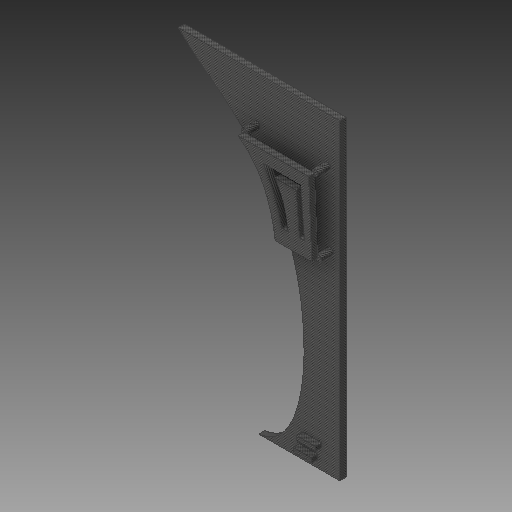
# Autodesk Inventor part: Part2 new side frame
Saved by Autodesk Inventor 2018 (Build 220112000, 112)
## iProperties
Created: 2021-03-13
Part Number: Part2 new side frame
Material: CFRP
Document SubType Name: Modeling
Designer: Abhig
Density: 1.43 g/cm^3
Appearance: Carbon Fiber
Author: Abhig
Autodesk Inventor part; units mm, degrees
ref_plane "YZ Plane" through (0, 0, 0) normal (1, 0, 0) x (0, 1, 0)
ref_plane "XZ Plane" through (0, 0, 0) normal (0, 1, 0) x (-1, 0, 0)
ref_plane "XY Plane" through (0, 0, 0) normal (0, 0, 1) x (1, 0, 0)
sketch "Sketch1" plane through (0, 0, 0) normal (0, 0, 1) x (1, 0, 0)
  line L0 (0, 226.8926) -> (200, 226.8926)
  line L1 (200, 226.8926) -> (200, -273.1074)
  line L2 (200, -273.1074) -> (70.0106, -273.1074)
  spline S0 degree 4 poles (0, 177.3413) (126.203, 79.0594) (154.2664, -10.2822) (176.0066, -260.8084) (70.0106, -273.1074) knots 0 0 0 0 0 1 1 1 1 1
  spline S1 degree 2 poles (0, 177.3413) (-36.5043, 204.7595) (-58.7785, 226.8926) knots 0 0 0 1 1 1
  line L3 (-58.7785, 226.8926) -> (0, 226.8926)
  point P0 (0, 0)
  point P1 (99.9997, 63.7426)
  point P2 (140.6791, -78.917)
  point P3 (126.8096, -220.2554)
  point P4 (-35.664, 205.7436)
  constraints: 8 end point, 2 horizontal, 1 parallel, 1 perpendicular, 10 other
extrude "Extrusion1" add sketch "Sketch1" along normal blind 10
sketch "Sketch2" plane through (0, 0, 10) normal (0, 0, 1) x (1, 0, 0)
  circle A0 centre (66.8612, 154.6625) radius 5
  circle A1 centre (180.0109, 154.6625) radius 5
  circle A2 centre (185.0109, 38.5738) radius 5
  circle A3 centre (126.375, 38.5738) radius 5
  point P0 (0, 0)
  dimension "d5" = 10
  dimension "d6" = 10
  dimension "d7" = 10
  dimension "d8" = 10
  constraints: 4 centre point
  measures "d5" diameter of A0
  measures "d6" diameter of A1
  measures "d7" diameter of A2
  measures "d8" diameter of A3
extrude "Extrusion2" add sketch "Sketch2" along normal blind 20
sketch "Sketch3" plane through (180.0109, 154.6625, 30) normal (0, 0, 1) x (1, 0, 0)
  circle A0 centre (-113.1497, 0) radius 5 projected
  circle A1 centre (0, 0) radius 5 projected
  line L0 (-113.1497, 0) -> (0, 0)
  circle A2 centre (5, -116.0887) radius 5 projected
  line L1 (0, 0) -> (5, -116.0887)
  circle A3 centre (-53.6359, -116.0887) radius 5 projected
  line L2 (5, -116.0887) -> (-53.6359, -116.0887)
  spline S0 degree 2 poles (-113.1497, 0) (-63.3738, -35.791) (-53.6359, -116.0887) knots 0 0 0 1 1 1
  point P0 (-180.0109, -154.6625)
  point P1 (-75.6781, -42.6148)
  constraints: 6 end point, 1 horizontal, 3 other
extrude "Extrusion3" add sketch "Sketch3" along normal blind 10 contours L0 A1 L1 A2 L2 A3 S0 A0 | A0 S0 L0 | L0 L1 A1 | A3 L2 S0 | L1 L2 A2 picked at (-110.3004, -1.6927) picked at (-1.6834, -2.8514) picked at (-53.6623, -112.78) picked at (1.7062, -115.7278)
sketch "Sketch4" plane through (180.0109, 154.6625, 40) normal (0, 0, 1) x (1, 0, 0)
  line L0 (-72.7391, -18.3685) -> (-12.7391, -18.3685)
  line L1 (-12.7391, -18.3685) -> (-6.5901, -92.1125)
  spline S0 degree 2 poles (-72.7391, -18.3685) (-51.5746, -50.5042) (-42.859, -93.2077) knots 0 0 0 1 1 1
  line L2 (-14.6388, -92.7837) -> (-19.9394, -29.2142)
  line L3 (-19.9394, -29.2142) -> (-55.1054, -29.2142)
  spline S1 degree 2 poles (-55.1054, -29.2142) (-38.2895, -49.2242) (-32.7381, -93.2077) knots 0 0 0 1 1 1
  line L4 (-42.859, -93.2077) -> (-32.7381, -93.2077)
  line L5 (-14.6388, -92.7837) -> (-6.5901, -92.1125)
  point P0 (-180.0109, -154.6625)
  point P1 (-55.1635, -51.9626)
  point P2 (-42.687, -50.9557)
  dimension "d13" = 60
  dimension "d14" = 74
  constraints: 12 end point, 3 horizontal, 1 perpendicular, 6 other
  measures "d13" distance of L0.start L0.end
  measures "d14" distance of L0.end L1.end
extrude "Extrusion4" cut sketch "Sketch4" against normal blind 10
sketch "Sketch6" plane through (0, 0, 10) normal (0, 0, 1) x (1, 0, 0)
  line L0 (135.0053, -253.8522) -> (165.0053, -253.8522)
  line L1 (165.0053, -253.8522) -> (165.0053, -260.8522)
  line L2 (165.0053, -260.8522) -> (135.0053, -260.8522)
  line L3 (135.0053, -260.8522) -> (135.0053, -253.8522)
  line L4 (141.0698, -234.749) -> (171.0698, -234.749)
  line L5 (171.0698, -234.749) -> (171.0698, -241.749)
  line L6 (171.0698, -241.749) -> (141.0698, -241.749)
  line L7 (141.0698, -241.749) -> (141.0698, -234.749)
  point P0 (0, 0)
  dimension "d22" = 30
  dimension "d23" = 7
  dimension "d24" = 30
  dimension "d25" = 7
  constraints: 16 end point, 4 parallel, 2 horizontal, 2 perpendicular
  measures "d22" distance of L1.end L2.end
  measures "d23" distance of L0.end L1.end
  measures "d24" distance of L5.end L6.end
  measures "d25" distance of L4.end L5.end
extrude "Extrusion6" add sketch "Sketch6" along normal blind 10
sketch "Sketch8" plane through (0, 0, 0) normal (0, 0, -1) x (-1, 0, 0)
  circle A0 centre (-180.0109, 154.6625) radius 5 projected
  circle A1 centre (-180.0109, 154.6625) radius 5
  line L0 (-180.0109, 154.6625) -> (-154.3956, -221.4322) construction
  circle A2 centre (-154.3956, -221.4322) radius 5
  point P0 (0, 0)
  dimension "d32" = 10
  dimension "d33" = 376.966
  dimension "d34" = 10
  constraints: 2 centre point, 2 coincident, 2 end point
  measures "d32" diameter of A1
  measures "d33" distance of L0.start L0.end
  measures "d34" diameter of A2
extrude "Extrusion8" add sketch "Sketch8" along normal blind 10
body "Solid1"
